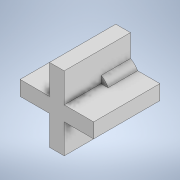
# Autodesk Inventor part: 2xxx_Rx_Coil_Winder_MPSv2_v1
Saved by Autodesk Inventor 2021 (Build 250183000, 183)
## iProperties
Created: 2020-09-17
Part Number: 2xxx_Rx_Coil_Winder_MPSv2_v1
Material: Generic
Document SubType Name: Modeling
Designer: Admin
Density: 1 g/cm^3
Appearance: Default
Author: Admin
Autodesk Inventor part; units mm, degrees
ref_plane "YZ Plane" through (0, 0, 0) normal (1, 0, 0) x (0, 1, 0)
ref_plane "XZ Plane" through (0, 0, 0) normal (0, 1, 0) x (-1, 0, 0)
ref_plane "XY Plane" through (0, 0, 0) normal (0, 0, 1) x (1, 0, 0)
sketch "Sketch1" plane through (0, 0, 0) normal (0, 0, 1) x (1, 0, 0)
  circle A0 centre (0, 0) radius 8.4
  circle A1 centre (0, 0) radius 11
  line L0 (9.5093, -0.878) -> (0, 0)
  line L1 (0, 0) -> (9.5093, 0.8821)
  line L2 (9.5093, 0.8821) -> (9.5093, -0.878)
  line L3 (0, 0) -> (-9.5093, 0.8821)
  line L4 (-9.5093, 0.8821) -> (-9.5093, -0.878)
  line L5 (-9.5093, -0.878) -> (0, 0)
  point P0 (8.3644, -0.7723)
  point P1 (-8.3644, -0.7723)
  point P2 (-8.3641, 0.7759)
  point P3 (8.3641, 0.7759)
  dimension "d0" = 16.8
  dimension "d1" = 22
  constraints: 12 end point, 2 centre point, 2 coincident, 1 vertical
  measures "d0" diameter of A0
  measures "d1" diameter of A1
extrude "Extrusion1" add sketch "Sketch1" along normal blind 15
sketch "Sketch2" plane through (0, 0, 15) normal (0, 0, 1) x (1, 0, 0)
  circle A0 centre (0, 0) radius 11
  constraints: 1 centre point, 1 coincident
extrude "Extrusion2" add sketch "Sketch2" along normal blind 5
sketch "Sketch3" plane through (0, 0, 20) normal (0, 0, 1) x (1, 0, 0)
  line L0 (-5, 5) -> (5, 5)
  line L1 (5, 5) -> (5, -5)
  line L2 (5, -5) -> (-5, -5)
  line L3 (-5, -5) -> (-5, 5)
  line L4 (-5, 5) -> (5, -5) construction
  line L5 (5, 5) -> (-5, -5) construction
  point P0 (0, 0)
  dimension "d6" = 10
  dimension "d7" = 10
  constraints: 12 end point, 2 midpoint, 2 parallel, 1 horizontal, 1 perpendicular
  measures "d6" distance of L1.end L2.end
  measures "d7" distance of L0.end L1.end
extrude "Extrusion3" add sketch "Sketch3" along normal blind 25
sketch "Sketch4" plane through (-5, 5, 20) normal (0, 1, 0) x (1, 0, 0)
  point P0 (5, 20)
sketch "Sketch5" plane through (-5, 5, 20) normal (0, 1, 0) x (1, 0, 0)
  line L0 (10, 0) -> (0, 0) projected
  line L1 (0, -25) -> (10, -25) projected
  line L2 (0, 0) -> (10, 0)
  line L3 (10, 0) -> (10, -25)
  line L4 (10, -25) -> (0, -25)
  line L5 (0, -25) -> (0, 0)
  point P0 (5, 20)
  constraints: 8 end point, 2 parallel, 1 horizontal, 1 perpendicular
sketch "Sketch6" plane through (5, -5, 20) normal (1, 0, 0) x (0, 0, -1)
  line L0 (0, 10) -> (0, 0) projected
  line L1 (0, 0) -> (-25, 0) projected
  line L2 (0, 10) -> (-25, 10)
  line L3 (-25, 10) -> (-25, 0)
  line L4 (-25, 0) -> (0, 0)
  line L5 (0, 0) -> (0, 10)
  point P0 (20, 5)
  constraints: 8 end point, 2 parallel, 1 horizontal, 1 perpendicular
extrude "Extrusion4" add sketch "Sketch6" along normal blind 20
extrude "Extrusion5" add sketch "Sketch5" along normal blind 20
mirror "Mirror1" about plane through (0, 0, 0) normal (0, 1, 0) of "Extrusion4", "Extrusion5"
mirror "Mirror2" about plane through (0, 0, 0) normal (1, 0, 0) of "Extrusion4"
sketch "Sketch7" plane through (25, 5, 20) normal (0, 0, -1) x (-1, 0, 0)
  line L0 (0, 0) -> (0, -10) projected
  arc A0 (20, 4.798) -> (15.202, 0) centre (25, -5) ccw projected
  line L1 (0, -10) -> (15.202, -10)
  line L2 (15.202, -10) -> (15.202, 0)
  line L3 (15.202, 0) -> (0, 0)
  line L4 (0, 0) -> (0, -10)
  arc A1 (15.202, 0) -> (15.202, -10) centre (25, -5) ccw projected
  circle A2 centre (25, -5) radius 11
  line L5 (20, -10) -> (20, -30) projected
  line L6 (30, -30) -> (30, -10) projected
  line L7 (20, -30) -> (30, -30)
  line L8 (30, -30) -> (30, -14.798)
  line L9 (30, -14.798) -> (20, -14.798)
  line L10 (20, -14.798) -> (20, -30)
  line L11 (30, 0) -> (30, 20) projected
  arc A3 (30, 4.798) -> (20, 4.798) centre (25, -5) ccw projected
  line L12 (30, 20) -> (20, 20)
  line L13 (20, 20) -> (20, 4.798)
  line L14 (20, 4.798) -> (30, 4.798)
  line L15 (30, 4.798) -> (30, 20)
  line L16 (30, 0) -> (50, 0) projected
  arc A4 (34.798, -10) -> (34.798, 0) centre (25, -5) ccw projected
  line L17 (50, 0) -> (34.798, 0)
  line L18 (34.798, 0) -> (34.798, -10)
  line L19 (34.798, -10) -> (50, -10)
  line L20 (50, -10) -> (50, 0)
  point P0 (30, 4.798)
  constraints: 32 end point, 8 parallel, 4 horizontal, 4 perpendicular, 2 point on circle, 1 centre point, 1 coincident, 1 point on line
extrude "Extrusion6" add sketch "Sketch7" along normal blind 20 contours L3 A1 L1 L0 | L13 L12 L11 A2 | A2 L6 L7 L5 | L16 L20 L19 A2
body "Solid1"
